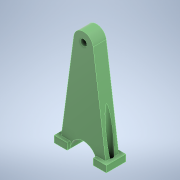
# Autodesk Inventor part: 连杆
Saved by Autodesk Inventor 2022 (Build 260153000, 153)
## iProperties
Created: 2023-02-21
Part Number: 连杆
Material: 常规
Document SubType Name: Modeling
Designer: 李承轩
Density: 1 g/cm^3
Appearance: 平滑 - 深森林绿
Author: 李承轩
Autodesk Inventor part; units mm, degrees
ref_plane "YZ Plane" through (0, 0, 0) normal (1, 0, 0) x (0, 1, 0)
ref_plane "XZ Plane" through (0, 0, 0) normal (0, 1, 0) x (-1, 0, 0)
ref_plane "XY Plane" through (0, 0, 0) normal (0, 0, 1) x (1, 0, 0)
sketch "草图1" plane through (0, 0, 0) normal (0, 0, 1) x (1, 0, 0)
  circle A0 centre (0, 0) radius 20 projected
  circle A1 centre (0, 0) radius 35
  line L0 (-35, 0) -> (35, 0)
  point P0 (-20, 0)
  point P1 (20, 0)
  dimension "d0" = 70
  dimension "d1" = 70
  constraints: 2 end point, 2 point on circle, 1 centre point, 1 coincident, 1 horizontal
  measures "d0" diameter of A1
  measures "d1" distance of L0.start L0.end
extrude "拉伸1" add sketch "草图1" along normal mid plane 20 contours A0 L0 A1 picked at (29.7075, 2.5961)
sketch "草图2" plane through (0, 0, 0) normal (0, 0, 1) x (1, 0, 0)
  arc A0 (20, 0) -> (-20, 0) centre (0, 0) ccw projected
  line L0 (-20, 0) -> (-40, 0)
  line L1 (-40, 0) -> (-40, 10)
  line L2 (-40, 10) -> (-20, 10)
  line L3 (-20, 10) -> (-20, 0)
  line L4 (35, 0) -> (20, 0) projected
  line L5 (20, 0) -> (40, 0)
  line L6 (40, 0) -> (40, 10)
  line L7 (40, 10) -> (20, 10)
  line L8 (20, 10) -> (20, 0)
  dimension "d4" = 20
  dimension "d5" = 10
  dimension "d6" = 20
  dimension "d7" = 10
  constraints: 16 end point, 4 parallel, 2 horizontal, 2 perpendicular
  measures "d4" distance of L1.end L2.end
  measures "d5" distance of L0.end L1.end
  measures "d6" distance of L7.end L6.end
  measures "d7" distance of L6.end L5.end
extrude "拉伸2" add sketch "草图2" along normal mid plane 30
sketch "草图3" plane through (0, 0, 0) normal (0, 0, 1) x (1, 0, 0)
  circle A0 centre (0, 150) radius 15
  line L0 (-20, 10) -> (-33.541, 10) projected
  arc A1 (33.541, 10) -> (-33.541, 10) centre (0, 0) ccw projected
  line L1 (33.541, 10) -> (20, 10) projected
  line L2 (20, 10) -> (20, 0) projected
  arc A2 (20, 0) -> (-20, 0) centre (0, 0) ccw projected
  line L3 (-20, 0) -> (-20, 10) projected
  circle A3 centre (0, 0) radius 35
  line L4 (-14.8661, 152) -> (-34.6875, 4.6667)
  line L5 (0, 0) -> (0, 98.8257)
  line L6 (14.8661, 152) -> (34.6875, 4.6667)
  dimension "d10" = 30
  dimension "d11" = 150
  constraints: 6 end point, 2 symmetric about line, 1 coincident, 1 tangent, 1 vertical, 1 vertical alignment, 8 other
  measures "d11" distance of point (0, 0) point (0, 150)
extrude "拉伸3" add sketch "草图3" along normal mid plane 20 contours A0 | A0 L6 A3 A1 L4
sketch "草图4" plane through (0, 0, 10) normal (0, 0, 1) x (1, 0, 0)
  arc A0 (14.8661, 152) -> (-14.8661, 152) centre (0, 150) ccw projected
  point P0 (0, 0)
  constraints: 1 coincident
hole "孔1" at (0, 150, 10) direction (0, 0, -1) diameter 10 end through all
sketch "草图5" plane through (-40, 0, 15) normal (0, -1, 0) x (1, 0, 0)
  line L0 (20, -5) -> (20, 0) construction
  line L1 (0, 0) -> (20, 0) construction
  line L2 (0, -30) -> (0, 0) construction
  line L3 (20, -30) -> (0, -30) construction
  line L4 (20, -30) -> (20, -25) construction
  line L5 (20, -5) -> (20, -25) construction
  point P0 (40, -15)
  point P1 (10, -15)
  point P2 (0, -15)
  point P3 (10, -30)
  constraints: 2 midpoint, 1 horizontal alignment, 1 vertical alignment
hole "孔2" at (-30, 0, 0) direction (0, 1, 0) diameter 10 end through all
mirror "镜像1" about plane through (0, 0, 0) normal (1, 0, 0) of "孔2"
